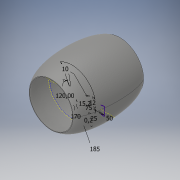
# Autodesk Inventor part: Form
Saved by Autodesk Inventor 2018.3 (Build 223284000, 284)
## iProperties
Created: 2018-07-22
Part Number: Form
Material: Generisch
Document SubType Name: Modeling
Designer: JochenAlt
Density: 1 g/cm^3
Appearance: Textur - grau
Author: JochenAlt
Autodesk Inventor part; units mm, degrees
ref_plane "YZ Plane" through (0, 0, 0) normal (1, 0, 0) x (0, 1, 0)
ref_plane "XZ Plane" through (0, 0, 0) normal (0, 1, 0) x (-1, 0, 0)
ref_plane "XY Plane" through (0, 0, 0) normal (0, 0, 1) x (1, 0, 0)
sketch "Skizze3" plane through (0, 0, 0) normal (0, 0, 1) x (1, 0, 0)
  line L0 (0, 257.2165) -> (0, -229.5361) construction
  line L1 (-127.2, 0) -> (203.2, 0) construction
  line L2 (92, 185) -> (90, 185)
  circle A0 centre (0, 0) radius 80 construction
  circle A1 centre (0, -80) radius 80 construction
  line L3 (83, -80) -> (85, -80)
  line L4 (83, -80) -> (124.4964, -36.286) construction
  line L5 (124.4964, 136.5571) -> (90, 185) construction
  spline S0 degree 3 poles (83, -80) (124.4964, -36.286) (124.4964, 136.5571) (90, 185) knots 1 1 1 1 2 2 2 2
  line L6 (92, 185) -> (126.4964, 136.5571) construction
  line L7 (126.4964, -36.286) -> (85, -80) construction
  spline S1 degree 3 poles (92, 185) (126.4964, 136.5571) (126.4964, -36.286) (85, -80) knots 1 1 1 1 2 2 2 2
  line L8 (154, 101.6438) -> (156, 101.6438) construction
  line L9 (154, 101.6438) -> (156, 101.6438) construction
  line L10 (126.4964, 136.5571) -> (126.4964, -36.286) construction
  line L11 (124.4964, -36.286) -> (124.4964, 136.5571) construction
  line L12 (57.5472, 55.5727) -> (101.7866, 98.2942) construction
  line L13 (57.5472, -24.4273) -> (101.7866, 18.2942) construction
  circle A2 centre (101.7866, 18.2942) radius 8.5 construction
  circle A3 centre (101.7866, 98.2942) radius 8.5 construction
  line L14 (83, -80) -> (80, -80) construction
  line L15 (110.2514, 17.5216) -> (113.239, 17.2489) construction
  line L16 (110.2516, 99.0643) -> (113.2393, 99.3361) construction
  line L17 (0, 125) -> (108, 125) construction
  line L18 (108, 125) -> (109.9737, 125.3234) construction
  point P0 (90, 149.8145)
  dimension "d13" = 160
  dimension "d108" = 17
  dimension "d7" = 185
  dimension "d11" = 2
  dimension "d14" = 80
  dimension "d15" = 90
  dimension "d18" = 2
  dimension "d19" = 2
  dimension "d105" = 2
  dimension "d106" = 61.5
  dimension "d107" = 46
  dimension "d110" = 3
  dimension "d111" = 3
  dimension "d112" = 3
  dimension "d113" = 108
  dimension "d114" = 125
  dimension "d115" = 2
  constraints: 22 end point, 6 parallel, 5 horizontal, 4 point on line, 2 coincident, 2 point on circle, 1 centre point, 1 collinear, 1 line through centre, 1 vertical, 24 other
  measures "d7" distance between parallel lines of L1 L2
  measures "d11" distance of L2.start L2.end
  measures "d14" distance of A1.centre point (0, 0)
  measures "d15" distance from line of L0 L2.end
  measures "d18" distance of L3.end L3.start
  measures "d19" distance of L8.start L8.end
  measures "d105" distance between parallel lines of L10 L11
  measures "d106" distance of L12.start L12.end
  measures "d107" angle of L0 L12
  measures "d110" distance of L3.start L14.end
  measures "d111" distance of L15.start L15.end
  measures "d112" distance of L16.start L16.end
  measures "d113" distance of L17.start L17.end
  measures "d114" distance between parallel lines of L17 L1
  measures "d115" distance of L17.end L18.end
revolve "Umdrehung1" add sketch "Skizze3" angle 360 about axis through (0, 0, 0) along (0, -1, 0)
sketch "Skizze6" plane through (0, 0, 0) normal (1, 0, 0) x (0, 1, 0)
  line L0 (-36, 0) -> (216, 0) construction
  line L1 (0, 126) -> (0, -126) construction
  line L2 (159, 25) -> (159, -25)
  line L3 (169, 25) -> (159, 25)
  line L4 (159, -25) -> (169, -25)
  line L5 (169, -25) -> (169, 25)
  line L6 (185, 90) -> (185, -90) projected
  point P0 (0, 0)
  point P1 (185, 0)
  dimension "d35" = 50
  dimension "d49" = 16
  dimension "d51" = 10
  constraints: 8 end point, 2 vertical, 1 horizontal, 1 parallel, 1 other
  measures "d35" distance of L2.start L2.end
  measures "d49" distance between parallel lines of L6 L5
  measures "d51" distance of L2.end L4.end
extrude "Extrusion4" add sketch "Skizze6" along normal up to next separate body
sketch "Skizze7" plane through (0, 0, 0) normal (0, 1, 0) x (-1, 0, 0)
  arc A0 (-91.6741, 12.3333) -> (-91.6741, -12.3333) centre (0, 0) ccw
  circle A1 centre (-75, 0) radius 7.6
  line L0 (-73.6667, -9.9107) -> (-91.6741, -12.3333)
  line L1 (-73.6667, 9.9107) -> (-91.6741, 12.3333)
  line L2 (-92, 0) -> (-117.0578, 0) construction
  arc A2 (-73.6667, -9.9107) -> (-73.6667, 9.9107) centre (-75, 0) ccw
  circle A3 centre (-75, 0) radius 6.6
  line L3 (-91.6741, -12.3333) -> (-125, -16.8168)
  line L4 (-91.6741, 12.3333) -> (-125, 16.8168)
  line L5 (-125, -16.8168) -> (-125, 16.8168)
  line L6 (-84.6958, 9.3765) -> (-84.4291, 11.3586) construction
  line L7 (0, 0) -> (-44.9, -77.7691) construction
  line L8 (0, 0) -> (-44.9, 77.7691) construction
  arc A4 (-44.9, 77.7691) -> (-44.9, -77.7691) centre (0, 0) ccw
  arc A5 (-32.4, 56.1184) -> (-32.4, -56.1184) centre (0, 0) ccw
  line L9 (-44.9, -77.7691) -> (-32.4, -56.1184)
  line L10 (-44.9, 77.7691) -> (-32.4, 56.1184)
  line L11 (-168, 0) -> (133, 0) construction
  circle A6 centre (0, 0) radius 85 construction
  circle A7 centre (0, 0) radius 90 construction
  point P0 (-90, 0)
  dimension "d32" = 185
  dimension "d40" = 15.2
  dimension "d50" = 75
  dimension "d52" = 10
  dimension "d53" = 1
  dimension "d56" = 50
  dimension "d67" = 2
  dimension "d72" = 25
  dimension "d101" = 170
  dimension "d103" = 120
  dimension "d116" = 0.2
  constraints: 20 end point, 8 point on circle, 7 centre point, 6 coincident, 5 point on line, 2 collinear, 2 tangent, 1 horizontal alignment, 1 perpendicular, 1 vertical, 2 other
  measures "d32" diameter of A0
  measures "d40" diameter of A1
  measures "d50" distance of A1.centre point (0, 0)
  measures "d52" radius of A2
  measures "d53" radial gap between concentric circles of A3 A1
  measures "d56" distance from line of L5 A1.centre
  measures "d67" distance of L6.start L6.end
  measures "d72" radial gap between concentric circles of A4 A5
  measures "d101" diameter of A6
  measures "d103" angle of L7 L8
extrude "Extrusion5" cut sketch "Skizze7" along normal through all both and the other way through all contours L1 A4 L0 A0 | A0 L3 L5 L4 | L1 A2 L0 A4 keep common part bodies 2
extrude "Extrusion8" add sketch "Skizze7" along normal blind 1 from surface at 159 contours A1 bodies 2
extrude "Extrusion9" add sketch "Skizze7" along normal blind 1 from surface at 159 contours A1 bodies 2
pattern_circular "Runde Anordnung2" count 3 over 360 about axis through (0, -10, 0) along (0, 1, 0) bodies 2
combine bodies "Kombinieren2" operation type add bodies to combine 2 1
extrude "Extrusion10" add sketch "Skizze7" against normal blind 1 from surface at 185 separate body contours A4 L10 A5 L9 L0 A2 L1 | L1 A2 L0 A4 | A1
extrude "Extrusion11" add sketch "Skizze7" against normal blind 4 from surface at 184 contours A4 L10 A5 L9 L0 A2 L1 | L1 A2 L0 A4 bodies 3
pattern_circular "Runde Anordnung3" count 3 over 360 about axis through (0, -10, 0) along (0, 1, 0) of "Extrusion10", "Extrusion11" bodies 3
equation "\"d14\" = 0.5 * d13"
equation "\"d18\" = d17"
equation "\"d16\" = d11"
equation "\"d17\" = d16"
